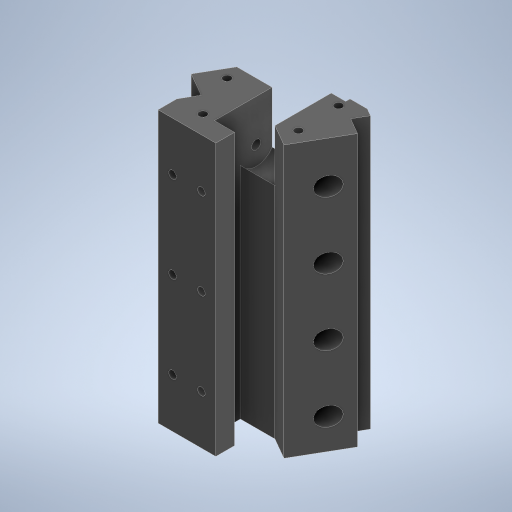
# Autodesk Inventor part: rail_base
Saved by Autodesk Inventor 2024.1 (Build 281209000, 209)
## iProperties
Created: 2025-01-17
Part Number: rail_base
Material: 一般
Document SubType Name: Modeling
Designer: hibik
Density: 1 g/cm^3
Appearance: 既定
Author: hibik
Autodesk Inventor part; units mm, degrees
ref_plane "YZ Plane" through (0, 0, 0) normal (1, 0, 0) x (0, 1, 0)
ref_plane "XZ Plane" through (0, 0, 0) normal (0, 1, 0) x (-1, 0, 0)
ref_plane "XY Plane" through (0, 0, 0) normal (0, 0, 1) x (1, 0, 0)
sketch "スケッチ1" plane through (0, 0, 0) normal (0, 1, 0) x (-1, 0, 0)
  line L0 (0, 0) -> (-19.1969, -33.25)
  line L1 (0, 0) -> (30, 0) construction
  line L2 (30, 0) -> (30, -18)
  line L3 (30, -18) -> (18.453, -38)
  line L4 (18.453, -38) -> (-10.9697, -38)
  line L5 (-10.9697, -38) -> (-19.1969, -33.25)
  line L6 (30, -1.5) -> (-0.866, -1.5)
  line L7 (25, -1.5) -> (5, -1.5)
  line L8 (5, -1.5) -> (5, -8)
  line L9 (5, -8) -> (25, -8) construction
  line L10 (25, -8) -> (25, -1.5)
  line L11 (30, -18) -> (21.9199, -13.3349)
  line L12 (21.9199, -13.3349) -> (25, -8)
  line L13 (30, -10.5) -> (25.6699, -8) construction
  line L14 (25.6699, -8) -> (22.4223, -13.625) construction
  line L15 (22.4223, -13.625) -> (26.7524, -16.125) construction
  line L16 (26.7524, -16.125) -> (30, -10.5) construction
  line L17 (5, -8) -> (12, -8)
  line L18 (12, -8) -> (12, -17)
  line L19 (12, -17) -> (5, -17)
  line L20 (5, -17) -> (5, -8) construction
  line L21 (5, -17) -> (0, -17)
  line L22 (0, -17) -> (-7.3612, -12.75)
  line L23 (0, -38) -> (0, -28)
  line L24 (0, -28) -> (24.2265, -28)
  line L25 (-13.5677, -36.5) -> (-11.0677, -32.1699)
  line L26 (-11.0677, -32.1699) -> (-16.6969, -28.9199)
  line L27 (0, -38) -> (-5, -38)
  line L28 (-5, -38) -> (-5, -36.5)
  line L29 (-5, -36.5) -> (0, -36.5)
  line L30 (0, -36.5) -> (0, -38)
  point P0 (-5, -38)
  point P1 (0, -36.5)
  dimension "d0" = 60
  dimension "d1" = 30
  dimension "d4" = 9.5
  dimension "d5" = 1.5
  dimension "d6" = 5
  dimension "d7" = 5
  dimension "d8" = 6.5
  dimension "d10" = 5
  dimension "d12" = 6.1602
  dimension "d14" = 9
  dimension "d15" = 7
  dimension "d18" = 10
  dimension "d19" = 10
  dimension "d20" = 6.5
  dimension "d21" = 5
  dimension "d22" = 3
  dimension "d23" = 5
  dimension "d24" = 1.5
  dimension "d26" = 38
  dimension "d27" = 18
  constraints: 62 end point, 11 parallel, 10 perpendicular, 10 point on line, 6 horizontal, 2 collinear, 2 vertical, 1 midpoint, 1 vertical alignment
  measures "d0" angle of L1 L0
  measures "d1" distance of L0.start L1.end
  measures "d4" distance from line of L4.end L0
  measures "d5" distance between parallel lines of L1 L6
  measures "d6" distance between parallel lines of L2 L10
  measures "d7" distance from line of L0.start L8
  measures "d8" distance of L9.end L7.start
  measures "d10" distance between parallel lines of L14 L16
  measures "d12" distance from line of L11 L9.end
  measures "d14" distance of L17.end L18.end
  measures "d15" distance of L18.end L19.end
  measures "d18" distance between parallel lines of L4 L24
  measures "d19" distance from line of L2.end L24
  measures "d20" distance between parallel lines of L0 L25
  measures "d21" distance between parallel lines of L5 L26
  measures "d22" distance from line of L4.end L25
  measures "d23" distance of L28.end L29.end
  measures "d24" distance of L27.end L28.end
  measures "d26" distance between parallel lines of L1 L4
  measures "d27" distance from line of L1 L2.end
extrude "押し出し1" add sketch "スケッチ1" along normal blind 94 contours L22 L21 L19 L18 L17 L8 L6 L10 L12 L11 L3 L24 L23 L29 L28 L4 L5 L25 L26 L0
sketch "スケッチ3" plane through (-12, 0, -8) normal (1, 0, 0) x (0, 0, -1)
  circle A0 centre (14.5, 79.5) radius 5.5
  line L0 (9, 0) -> (9, 94) projected
  line L1 (20, 0) -> (20, 94) projected
  line L2 (0, 94) -> (9, 94) projected
  line L3 (0, 94) -> (-6.5, 94) projected
  line L4 (-6.5, 94) -> (0, 94) projected
  line L5 (0, 94) -> (9, 94) projected
  line L6 (9, 94) -> (4.75, 94) projected
  line L7 (4.75, 94) -> (20.9199, 94) projected
  line L8 (20.9199, 94) -> (24.1699, 94) projected
  line L9 (24.1699, 94) -> (28.5, 94) projected
  line L10 (28.5, 94) -> (30, 94) projected
  line L11 (30, 94) -> (28.5, 94) projected
  line L12 (28.5, 94) -> (20, 94) projected
  line L13 (20, 94) -> (10, 94) projected
  line L14 (10, 94) -> (5.3349, 94) projected
  line L15 (5.3349, 94) -> (0, 94) projected
  circle A1 centre (14.5, 79.5) radius 6.5
  point P0 (-8, 0)
  point P1 (9, 79.5)
  point P2 (20, 79.5)
  point P3 (9, 82.9641)
  point P4 (20, 82.9641)
  dimension "d28" = 11
  dimension "d29" = 14.5
  dimension "d32" = 13
  constraints: 2 centre point, 2 tangent, 1 coincident
  measures "d28" diameter of A0
  measures "d29" distance from line of L2 A0.centre
  measures "d32" diameter of A1
extrude "押し出し2" cut sketch "スケッチ3" along normal up to surface (12 mm away)
sketch "スケッチ4" plane through (-12, 0, -8) normal (1, 0, 0) x (0, 0, -1)
  arc A0 (9, 76.0359) -> (20, 76.0359) centre (14.5, 79.5) ccw projected
  circle A1 centre (14.5, 79.5) radius 1.6
  point P0 (-8, 0)
  dimension "d33" = 3.2
  constraints: 1 centre point, 1 coincident
  measures "d33" diameter of A1
extrude "押し出し3" cut sketch "スケッチ4" against normal blind 8
sketch "スケッチ5" plane through (0, 0, -36.5) normal (-1, 0, 0) x (0, 0, 1)
  circle A0 centre (14, 79.5) radius 1.6 construction
  circle A1 centre (14, 79.5) radius 1.6
  line L0 (0, 0) -> (0, 94) projected
  circle A2 centre (14, 56.5) radius 1.6
  circle A3 centre (14, 33.5) radius 1.6
  circle A4 centre (14, 10.5) radius 1.6
  point P0 (36.5, 0)
  dimension "d36" = 3.2
  dimension "d39" = 23
  constraints: 4 centre point, 1 coincident, 1 vertical, 6 other
  measures "d36" diameter of A1
  measures "d39" distance of A1.centre A2.centre
extrude "押し出し4" cut sketch "スケッチ5" along normal through all both and the other way through all
ref_plane "作業平面1" through (-15, 0, -8) normal (1, 0, 0) x (0, 0, -1)
sketch "スケッチ6" plane through (-15, 0, -8) normal (1, 0, 0) x (0, 0, -1)
  circle A0 centre (14.5, 56.5) radius 1.6 projected
  circle A1 centre (14.5, 33.5) radius 1.6 projected
  circle A2 centre (14.5, 10.5) radius 1.6 projected
  line L0 (17.7909, 79.5) -> (16.1454, 76.65)
  line L1 (16.1454, 76.65) -> (12.8546, 76.65)
  line L2 (12.8546, 76.65) -> (11.2091, 79.5)
  line L3 (11.2091, 79.5) -> (12.8546, 82.35)
  line L4 (12.8546, 82.35) -> (16.1454, 82.35)
  line L5 (16.1454, 82.35) -> (17.7909, 79.5)
  line L6 (17.7909, 56.5) -> (16.1454, 53.65)
  line L7 (16.1454, 53.65) -> (12.8546, 53.65)
  line L8 (12.8546, 53.65) -> (11.2091, 56.5)
  line L9 (11.2091, 56.5) -> (12.8546, 59.35)
  line L10 (12.8546, 59.35) -> (16.1454, 59.35)
  line L11 (16.1454, 59.35) -> (17.7909, 56.5)
  line L12 (17.7909, 33.5) -> (16.1454, 30.65)
  line L13 (16.1454, 30.65) -> (12.8546, 30.65)
  line L14 (12.8546, 30.65) -> (11.2091, 33.5)
  line L15 (11.2091, 33.5) -> (12.8546, 36.35)
  line L16 (12.8546, 36.35) -> (16.1454, 36.35)
  line L17 (16.1454, 36.35) -> (17.7909, 33.5)
  line L18 (17.7909, 10.5) -> (16.1454, 7.65)
  line L19 (16.1454, 7.65) -> (12.8546, 7.65)
  line L20 (12.8546, 7.65) -> (11.2091, 10.5)
  line L21 (11.2091, 10.5) -> (12.8546, 13.35)
  line L22 (12.8546, 13.35) -> (16.1454, 13.35)
  line L23 (16.1454, 13.35) -> (17.7909, 10.5)
  circle A3 centre (14.5, 79.5) radius 1.6 projected
  point P0 (-8, 0)
  dimension "d47" = 5.7
  constraints: 48 end point, 4 coincident, 4 horizontal, 3 parallel, 52 other
  measures "d47" distance between parallel lines of L1 L4
extrude "押し出し5" cut sketch "スケッチ6" against normal through all contours A0 | A1 | A2 | L0 L1 L2 L3 L4 L5 | L6 L7 L8 L9 L10 L11 | L12 L13 L14 L15 L16 L17 | L18 L19 L20 L21 L22 L23 | A3
ref_plane "作業平面2" through (2, 0, -36.5) normal (-1, 0, 0) x (0, 0, 1)
sketch "スケッチ7" plane through (2, 0, -36.5) normal (-1, 0, 0) x (0, 0, 1)
  circle A0 centre (14, 79.5) radius 1.6 projected
  circle A1 centre (14, 56.5) radius 1.6 projected
  circle A2 centre (14, 33.5) radius 1.6 projected
  circle A3 centre (14, 10.5) radius 1.6 projected
  circle A4 centre (14, 79.5) radius 3.25
  circle A5 centre (14, 56.5) radius 1.6 projected
  circle A6 centre (14, 56.5) radius 3.25
  circle A7 centre (14, 33.5) radius 3.25
  circle A8 centre (14, 10.5) radius 3.25
  point P0 (36.5, 0)
  dimension "d51" = 6.5
  dimension "d52" = 6.5
  dimension "d53" = 6.5
  dimension "d54" = 6.5
  constraints: 4 centre point, 4 coincident
  measures "d51" diameter of A4
  measures "d52" diameter of A6
  measures "d53" diameter of A7
  measures "d54" diameter of A8
extrude "押し出し6" cut sketch "スケッチ7" against normal through all contours A0 | A1 | A2 | A3 | A4 | A6 | A7 | A8
sketch "スケッチ8" plane through (-25, 0, -1.5) normal (0, 0, 1) x (1, 0, 0)
  circle A0 centre (5, 77) radius 1.6 construction
  circle A1 centre (15, 77) radius 1.6 construction
  circle A2 centre (5, 47) radius 1.6 construction
  circle A3 centre (15, 47) radius 1.6 construction
  circle A4 centre (5, 17) radius 1.6 construction
  circle A5 centre (15, 17) radius 1.6 construction
  circle A6 centre (5, 77) radius 1.35
  circle A7 centre (15, 77) radius 1.35
  circle A8 centre (5, 47) radius 1.35
  circle A9 centre (15, 47) radius 1.35
  circle A10 centre (5, 17) radius 1.35
  circle A11 centre (15, 17) radius 1.35
  point P0 (25, 0)
  dimension "d59" = 2.7
  constraints: 6 centre point, 6 coincident, 5 equal radius
  measures "d59" diameter of A6
extrude "押し出し7" cut sketch "スケッチ8" against normal blind 5
ref_plane "作業平面3" through (0, 7, 0) normal (0, -1, 0) x (1, 0, 0)
sketch "スケッチ9" plane through (0, 7, 0) normal (0, -1, 0) x (1, 0, 0)
  line L0 (0, -38) -> (10.1, -38)
  line L1 (10.1, -38) -> (10.1, -30.8)
  line L2 (10.1, -30.8) -> (0, -30.8)
  line L3 (0, -30.8) -> (0, -38)
  line L4 (10.9697, -38) -> (-1, -38) projected
  point P0 (0, 0)
  point P1 (0, -36.5)
  dimension "d61" = 10.1
  dimension "d62" = 7.2
  constraints: 8 end point, 2 parallel, 1 collinear, 1 horizontal, 1 perpendicular, 1 point on line
  measures "d61" distance of L2.end L1.end
  measures "d62" distance of L1.end L0.end
extrude "押し出し8" cut sketch "スケッチ9" against normal blind 7.2
sketch "スケッチ11" plane through (0, 7, 0) normal (0, 1, 0) x (1, 0, 0)
  line L0 (5, 36.5) -> (5, 38) projected
  line L1 (5, 38) -> (0, 38)
  line L2 (0, 38) -> (0, 36.5)
  line L3 (0, 36.5) -> (5, 36.5)
  line L4 (5, 36.5) -> (5, 38)
  point P0 (0, 0)
  constraints: 8 end point, 2 parallel, 1 horizontal, 1 perpendicular
extrude "押し出し9" add sketch "スケッチ11" against normal up to surface (7 mm away)
sketch "スケッチ12" plane through (0, 14.2, 0) normal (0, -1, 0) x (1, 0, 0)
  line L0 (5, -36.5) -> (0, -36.5) projected
  line L1 (5, -38) -> (0, -38)
  line L2 (0, -38) -> (0, -36.5)
  line L3 (0, -36.5) -> (5, -36.5)
  line L4 (5, -36.5) -> (5, -38)
  point P0 (0, 0)
  constraints: 8 end point, 2 parallel, 1 horizontal, 1 perpendicular
extrude "押し出し10" add sketch "スケッチ12" against normal blind 10
sketch "スケッチ14" plane through (0, 0, 0) normal (0, -1, 0) x (1, 0, 0)
  circle A0 centre (5, -34) radius 1.6 projected
  point P0 (0, 0)
extrude "押し出し11" cut sketch "スケッチ14" against normal blind 30
sketch "スケッチ15" plane through (0, 0, 0) normal (0, -1, 0) x (1, 0, 0)
  circle A0 centre (5, -34) radius 1.6 projected
  circle A1 centre (5, -34) radius 2.5
  point P0 (0, 0)
  dimension "d71" = 5
  constraints: 1 centre point, 1 coincident
  measures "d71" diameter of A1
extrude "押し出し12" cut sketch "スケッチ15" against normal blind 4 contours A0 | A1
sketch "スケッチ16" plane through (0, 24.2, 0) normal (0, 1, 0) x (1, 0, 0)
  circle A0 centre (5, 34) radius 1.6 projected
  line L0 (3.3546, 36.85) -> (6.6454, 36.85)
  line L1 (6.6454, 36.85) -> (8.2909, 34)
  line L2 (8.2909, 34) -> (6.6454, 31.15)
  line L3 (6.6454, 31.15) -> (3.3546, 31.15)
  line L4 (3.3546, 31.15) -> (1.7091, 34)
  line L5 (1.7091, 34) -> (3.3546, 36.85)
  line L6 (8.2909, 34) -> (8.2909, 38)
  line L7 (1.7091, 34) -> (1.7091, 38)
  line L8 (8.2909, 38) -> (1.7091, 38)
  line L9 (5, 38) -> (0, 38) projected
  point P0 (0, 0)
  dimension "d74" = 5.7
  constraints: 18 end point, 2 horizontal, 2 vertical, 1 coincident, 1 collinear, 13 other
  measures "d74" distance between parallel lines of L3 L0
extrude "押し出し13" cut sketch "スケッチ16" against normal blind 4 contours A0 | L5 L7 L8 L6 L1 L0 | L0 L1 L2 L3 L4 L5
ref_plane "作業平面4" through (0, 14, 0) normal (0, -1, 0) x (1, 0, 0)
sketch "スケッチ17" plane through (0, 14, 0) normal (0, -1, 0) x (1, 0, 0)
  line L0 (-28.3519, -20.8546) -> (-29.3019, -19.2091) projected
  line L1 (-29.3019, -19.2091) -> (-28.3519, -20.8546) projected
  line L2 (-28.3519, -20.8546) -> (-26.4519, -24.1454) projected
  line L3 (-26.4519, -24.1454) -> (-25.5019, -25.7909) projected
  line L4 (-25.5019, -25.7909) -> (-26.4519, -24.1454) projected
  line L5 (-26.4519, -24.1454) -> (-28.3519, -20.8546) projected
  line L6 (-28.3519, -20.8546) -> (-29.3019, -19.2091) projected
  line L7 (-29.3019, -19.2091) -> (-28.3519, -20.8546) projected
  line L8 (-28.3519, -20.8546) -> (-26.4519, -24.1454) projected
  line L9 (-26.4519, -24.1454) -> (-25.5019, -25.7909) projected
  line L10 (-25.5019, -25.7909) -> (-26.4519, -24.1454) projected
  line L11 (-26.4519, -24.1454) -> (-28.3519, -20.8546) projected
  line L12 (-28.3519, -20.8546) -> (-29.3019, -19.2091) projected
  line L13 (-29.3019, -19.2091) -> (-28.3519, -20.8546) projected
  line L14 (-28.3519, -20.8546) -> (-26.4519, -24.1454) projected
  line L15 (-26.4519, -24.1454) -> (-25.5019, -25.7909) projected
  line L16 (-25.5019, -25.7909) -> (-26.4519, -24.1454) projected
  line L17 (-26.4519, -24.1454) -> (-28.3519, -20.8546) projected
  line L18 (-28.3519, -20.8546) -> (-29.3019, -19.2091) projected
  line L19 (-29.3019, -19.2091) -> (-28.3519, -20.8546) projected
  line L20 (-28.3519, -20.8546) -> (-26.4519, -24.1454) projected
  line L21 (-26.4519, -24.1454) -> (-25.5019, -25.7909) projected
  line L22 (-25.5019, -25.7909) -> (-26.4519, -24.1454) projected
  line L23 (-26.4519, -24.1454) -> (-28.3519, -20.8546) projected
  line L24 (-24.2265, -28) -> (-30, -18) projected
  line L25 (-24.2265, -28) -> (-30, -18) projected
  line L26 (-23.8301, -38.6865) -> (-29.0263, -41.6865)
  line L27 (-29.0263, -41.6865) -> (-39.0263, -24.366)
  line L28 (-39.0263, -24.366) -> (-33.8301, -21.366)
  line L29 (-33.8301, -21.366) -> (-23.8301, -38.6865)
  line L30 (-24.2265, -28) -> (-23.8301, -38.6865)
  line L31 (-33.8301, -21.366) -> (-29.5, -18.866)
  point P0 (0, 0)
  dimension "d78" = 1
  dimension "d79" = 20
  dimension "d80" = 11
  dimension "d81" = 6
  constraints: 12 end point, 3 parallel, 2 point on line, 1 perpendicular
  measures "d78" distance from line of L24.end L28
  measures "d79" distance between parallel lines of L26 L28
  measures "d80" distance between parallel lines of L24 L27
  measures "d81" distance between parallel lines of L27 L29
extrude "押し出し14" add sketch "スケッチ17" against normal blind 2
fillet "フィレット1" radius 3 1 edges at (-26.8632, 16, -23.433)
sketch "スケッチ18" plane through (5, 94, -36.5) normal (0, 0, -1) x (-1, 0, 0)
  circle A0 centre (2.5, -10) radius 1.6 projected
  circle A1 centre (2.5, -35) radius 1.6 projected
  circle A2 centre (2.5, -60) radius 1.6 projected
  circle A3 centre (2.5, -10) radius 1.35
  circle A4 centre (2.5, -35) radius 1.35
  circle A5 centre (2.5, -60) radius 1.35
  point P0 (5, -94)
  dimension "d85" = 2.7
  constraints: 3 centre point, 3 coincident, 2 equal radius
  measures "d85" diameter of A3
extrude "押し出し15" cut sketch "スケッチ18" against normal blind 5 contours A3 | A4 | A5
sketch "スケッチ19" plane through (0, 94, 0) normal (0, 1, 0) x (1, 0, 0)
  line L0 (2, 25.75) -> (14.8668, 25.75) projected
  circle A0 centre (5, 34) radius 1.6 projected
  circle A1 centre (5.5311, 19.5801) radius 1.6 projected
  circle A2 centre (-16, 8) radius 1.6 projected
  circle A3 centre (-22.5359, 22.9282) radius 1.6 projected
  line L1 (19.1969, 33.25) -> (10.9697, 38) projected
  line L2 (10.9697, 38) -> (10.9697, 39) projected
  line L3 (10.9697, 39) -> (-18.453, 39) projected
  line L4 (-18.453, 39) -> (-18.453, 38) projected
  line L5 (-18.453, 38) -> (-30, 18) projected
  line L6 (-30, 1.5) -> (0.866, 1.5) projected
  line L7 (0.866, 1.5) -> (19.1969, 33.25) projected
  circle A4 centre (5, 34) radius 1.35
  circle A5 centre (5.5311, 19.5801) radius 1.35
  circle A6 centre (-22.5359, 22.9282) radius 1.35
  circle A7 centre (-16, 8) radius 1.35
  line L8 (-30, 18) -> (-30, 1.5) projected
  point P0 (0, 0)
  dimension "d88" = 2.7
  dimension "d89" = 2.7
  dimension "d90" = 2.7
  dimension "d91" = 2.7
  constraints: 4 centre point, 4 coincident
  measures "d88" diameter of A4
  measures "d89" diameter of A5
  measures "d90" diameter of A6
  measures "d91" diameter of A7
extrude "押し出し16" cut sketch "スケッチ19" against normal blind 10 contours A4 | A5 | A6 | A7
ref_plane "作業平面5" through (0, 47, 0) normal (0, 1, 0) x (1, 0, 0)
mirror "ミラー1" about plane through (0, 47, 0) normal (0, 1, 0) of "押し出し16"
sketch "スケッチ20" plane through (0, 0, 0) normal (0, -1, 0) x (1, 0, 0)
  circle A0 centre (-6, -23) radius 1.35
  line L0 (0, -28) -> (-24.2265, -28) projected
  point P0 (0, 0)
  dimension "d95" = 2.7
  dimension "d96" = 5
  dimension "d97" = 6
  constraints: 1 centre point
  measures "d95" diameter of A0
  measures "d96" distance from line of L0 A0.centre
  measures "d97" horizontal distance of L0.start A0.centre
extrude "押し出し17" cut sketch "スケッチ20" against normal blind 10
ref_plane "作業平面6" through (-18, 0, -8) normal (-1, 0, 0) x (0, 0, 1)
sketch "スケッチ22" plane through (-18, 0, -8) normal (-1, 0, 0) x (0, 0, 1)
  circle A0 centre (-14.5, 79.5) radius 1.6 projected
  line L0 (-16.1454, 82.35) -> (-12.8546, 82.35) projected
  line L1 (-17.7909, 79.5) -> (-16.1454, 82.35) projected
  line L2 (-16.1454, 76.65) -> (-17.7909, 79.5) projected
  line L3 (-12.8546, 76.65) -> (-16.1454, 76.65) projected
  line L4 (-11.2091, 79.5) -> (-12.8546, 76.65) projected
  line L5 (-12.8546, 82.35) -> (-11.2091, 79.5) projected
  circle A1 centre (-14.5, 56.5) radius 1.6 projected
  line L6 (-16.1454, 59.35) -> (-12.8546, 59.35) projected
  line L7 (-17.7909, 56.5) -> (-16.1454, 59.35) projected
  line L8 (-16.1454, 53.65) -> (-17.7909, 56.5) projected
  line L9 (-12.8546, 53.65) -> (-16.1454, 53.65) projected
  line L10 (-11.2091, 56.5) -> (-12.8546, 53.65) projected
  line L11 (-12.8546, 59.35) -> (-11.2091, 56.5) projected
  circle A2 centre (-14.5, 33.5) radius 1.6 projected
  line L12 (-16.1454, 36.35) -> (-12.8546, 36.35) projected
  line L13 (-17.7909, 33.5) -> (-16.1454, 36.35) projected
  line L14 (-16.1454, 30.65) -> (-17.7909, 33.5) projected
  line L15 (-12.8546, 30.65) -> (-16.1454, 30.65) projected
  line L16 (-11.2091, 33.5) -> (-12.8546, 30.65) projected
  line L17 (-12.8546, 36.35) -> (-11.2091, 33.5) projected
  circle A3 centre (-14.5, 10.5) radius 1.6 projected
  line L18 (-16.1454, 13.35) -> (-12.8546, 13.35) projected
  line L19 (-17.7909, 10.5) -> (-16.1454, 13.35) projected
  line L20 (-16.1454, 7.65) -> (-17.7909, 10.5) projected
  line L21 (-12.8546, 7.65) -> (-16.1454, 7.65) projected
  line L22 (-11.2091, 10.5) -> (-12.8546, 7.65) projected
  line L23 (-12.8546, 13.35) -> (-11.2091, 10.5) projected
  line L24 (-10.7472, 10.5) -> (-12.6236, 7.25)
  line L25 (-12.6236, 7.25) -> (-16.3764, 7.25)
  line L26 (-16.3764, 7.25) -> (-18.2528, 10.5)
  line L27 (-18.2528, 10.5) -> (-16.3764, 13.75)
  line L28 (-16.3764, 13.75) -> (-12.6236, 13.75)
  line L29 (-12.6236, 13.75) -> (-10.7472, 10.5)
  line L30 (-10.7472, 33.5) -> (-12.6236, 30.25)
  line L31 (-12.6236, 30.25) -> (-16.3764, 30.25)
  line L32 (-16.3764, 30.25) -> (-18.2528, 33.5)
  line L33 (-18.2528, 33.5) -> (-16.3764, 36.75)
  line L34 (-16.3764, 36.75) -> (-12.6236, 36.75)
  line L35 (-12.6236, 36.75) -> (-10.7472, 33.5)
  line L36 (-10.7472, 79.5) -> (-12.6236, 76.25)
  line L37 (-12.6236, 76.25) -> (-16.3764, 76.25)
  line L38 (-16.3764, 76.25) -> (-18.2528, 79.5)
  line L39 (-18.2528, 79.5) -> (-16.3764, 82.75)
  line L40 (-16.3764, 82.75) -> (-12.6236, 82.75)
  line L41 (-12.6236, 82.75) -> (-10.7472, 79.5)
  line L42 (-10.7472, 56.5) -> (-12.6236, 53.25)
  line L43 (-12.6236, 53.25) -> (-16.3764, 53.25)
  line L44 (-16.3764, 53.25) -> (-18.2528, 56.5)
  line L45 (-18.2528, 56.5) -> (-16.3764, 59.75)
  line L46 (-16.3764, 59.75) -> (-12.6236, 59.75)
  line L47 (-12.6236, 59.75) -> (-10.7472, 56.5)
  point P0 (8, 0)
  dimension "d101" = 6.5
  constraints: 48 end point, 4 coincident, 4 horizontal, 3 parallel, 52 other
  measures "d101" distance between parallel lines of L37 L40
extrude "押し出し18" cut sketch "スケッチ22" along normal through all contours A0 | L0 L5 L4 L3 L2 L1 | A1 | L6 L11 L10 L9 L8 L7 | A2 | L12 L17 L16 L15 L14 L13 | A3 | L18 L23 L22 L21 L20 L19 | L24 L25 L26 L27 L28 L29 | L30 L31 L32 L33 L34 L35 | L36 L37 L38 L39 L40 L41 | L42 L43 L44 L45 L46 L47
equation "\"d52\" = d51"
equation "\"d53\" = d52"
equation "\"d54\" = d53"
